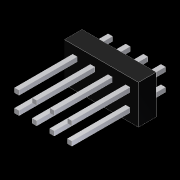
# Autodesk Inventor part: J23
Saved by Autodesk Inventor 2012 (Build 160160000, 160)
## iProperties
Company: Team 801
Created: 2009-08-01
Part Number: J23
Document SubType Name: Modeling
Designer: Jeffrey M
Density: 1 g/cm^3
Catalog Web Link: www.team801.org
Material: Default
Mass: 0.186649 g
Surface Area: 4.23741 cm^2
Volume: 0.186649 cm^3
Author: Jeffrey M
Autodesk Inventor part; units mm, degrees
ref_plane "YZ Plane" through (0, 0, 0) normal (1, 0, 0) x (0, 1, 0)
ref_plane "XZ Plane" through (0, 0, 0) normal (0, 1, 0) x (-1, 0, 0)
ref_plane "XY Plane" through (0, 0, 0) normal (0, 0, 1) x (1, 0, 0)
sketch "Sketch1" plane through (0, 0, 0) normal (0, 0, 1) x (1, 0, 0)
  line L0 (0, 5.588) -> (10.668, 5.588)
  line L1 (10.668, 5.588) -> (10.668, 0)
  line L2 (10.668, 0) -> (0, 0)
  line L3 (0, 0) -> (0, 5.588)
  line L4 (9.4615, 4.3815) -> (8.8265, 4.3815)
  line L5 (9.4615, 3.7465) -> (9.4615, 4.3815)
  line L6 (8.8265, 3.7465) -> (9.4615, 3.7465)
  line L7 (8.8265, 4.3815) -> (8.8265, 3.7465)
  constraints: 16 end point
extrude "Extrusion1" add sketch "Sketch1" against normal blind 2.54
extrude "Extrusion2" add sketch "Sketch1" along normal blind 8.382 contours L5 L6 L7 L4
extrude "Extrusion3" add sketch "Sketch1" against normal blind 5.08 contours L5 L6 L7 L4
pattern_linear "Rectangular Pattern1" count 4 spacing 2.54 along (-1, 0, 0) count 2 spacing 2.54 along (0, -1, 0) of "Extrusion3", "Extrusion2"
body "Solid1"
